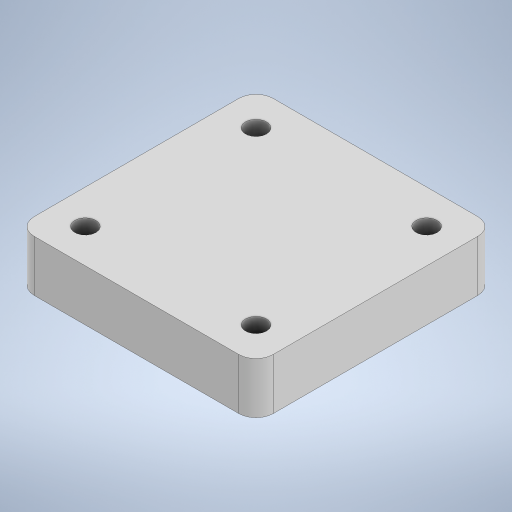
# Autodesk Inventor part: post_bottom
Saved by Autodesk Inventor 2024.3 (Build 283343000, 343)
## iProperties
Created: 2025-10-16
Part Number: post_bottom
Material: 일반
Document SubType Name: Modeling
Designer: joung
Density: 1 g/cm^3
Appearance: 기본값
Author: joung
Autodesk Inventor part; units mm, degrees
ref_plane "YZ Plane" through (0, 0, 0) normal (1, 0, 0) x (0, 1, 0)
ref_plane "XZ Plane" through (0, 0, 0) normal (0, 1, 0) x (-1, 0, 0)
ref_plane "XY Plane" through (0, 0, 0) normal (0, 0, 1) x (1, 0, 0)
sketch "스케치1" plane through (0, 0, 0) normal (0, 1, 0) x (-1, 0, 0)
  line L0 (25, 25) -> (-25, 25)
  line L1 (-25, 25) -> (-25, -25)
  line L2 (-25, -25) -> (25, -25)
  line L3 (25, -25) -> (25, 25)
  line L4 (25, 25) -> (-25, -25) construction
  line L5 (-25, 25) -> (25, -25) construction
  circle A0 centre (25, -25) radius 3.1
  circle A1 centre (25, 25) radius 3.1
  circle A2 centre (-25, 25) radius 3.1
  circle A3 centre (-25, -25) radius 3.1
  line L6 (-35, -30) -> (-35, 30)
  line L7 (-30, 35) -> (30, 35)
  line L8 (35, 30) -> (35, -30)
  line L9 (30, -35) -> (-30, -35)
  arc A4 (30, -35) -> (35, -30) centre (30, -30) ccw
  arc A5 (35, 30) -> (30, 35) centre (30, 30) ccw
  arc A6 (-30, 35) -> (-35, 30) centre (-30, 30) ccw
  arc A7 (-35, -30) -> (-30, -35) centre (-30, -30) ccw
  point P0 (0, 0)
  dimension "d0" = 50
  dimension "d1" = 50
  dimension "d2" = 6.2
  dimension "d5" = 360
  dimension "d7" = 10
  dimension "d8" = 5
  constraints: 20 end point, 8 centre point, 8 point on circle, 8 tangent, 4 parallel, 3 equal radius, 2 midpoint, 2 perpendicular, 1 coincident, 1 horizontal, 12 other
  measures "d0" distance of L2.end L1.end
  measures "d1" distance of L1.end L0.end
  measures "d2" diameter of A0
  measures "d7" distance between parallel lines of L1 L6
  measures "d8" radius of A4
extrude "돌출1" add sketch "스케치1" along normal blind 15 contours L0 A1 L3 A0 L2 A3 L1 A2 | L6 A6 L7 A5 L8 A4 L9 A7
